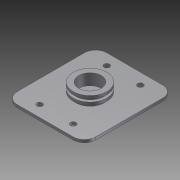
# Autodesk Inventor part: Rotation Base
Saved by Autodesk Inventor 2012 (Build 160160000, 160)
## iProperties
Created: 2011-10-21
Part Number: Rotation Base
Material: Aluminum-6061
Document SubType Name: Modeling
Designer: Tushar
Density: 2.71 g/cm^3
Mass: 90.9664 g
Surface Area: 227.283 cm^2
Volume: 33.5669 cm^3
Author: Tushar
Autodesk Inventor part; units mm, degrees
ref_plane "YZ Plane" through (0, 0, 0) normal (1, 0, 0) x (0, 1, 0)
ref_plane "XZ Plane" through (0, 0, 0) normal (0, 1, 0) x (-1, 0, 0)
ref_plane "XY Plane" through (0, 0, 0) normal (0, 0, 1) x (1, 0, 0)
sketch "Sketch2" plane through (0, 0, 0) normal (0, 1, 0) x (-1, 0, 0)
  line L0 (-44.45, 50.8) -> (44.45, 50.8)
  line L1 (44.45, 50.8) -> (44.45, -50.8)
  line L2 (44.45, -50.8) -> (-44.45, -50.8)
  line L3 (-44.45, -50.8) -> (-44.45, 50.8)
  point P0 (0, 0)
  dimension "d0" = 44.45
  dimension "d1" = 44.45
  dimension "d2" = 50.8
  dimension "d3" = 50.8
  constraints: 8 end point, 2 parallel, 1 horizontal, 1 perpendicular
  measures "d0" distance from line of L1 point (0, 0)
  measures "d1" distance from line of L3 point (0, 0)
  measures "d2" distance from line of L2 point (0, 0)
  measures "d3" distance from line of L0 point (0, 0)
extrude "Extrusion1" add sketch "Sketch2" along normal blind 3.175
fillet "Fillet1" radius 12.7 4 edges at (44.45, 1.5875, 50.8) (44.45, 1.5875, -50.8) (-44.45, 1.5875, 50.8) (-44.45, 1.5875, -50.8)
sketch "Sketch3" plane through (0, 3.175, 0) normal (0, 1, 0) x (1, 0, 0)
  line L0 (-44.45, -38.1) -> (-44.45, 38.1) projected
  line L1 (31.75, -50.8) -> (-31.75, -50.8) projected
  line L2 (44.45, 38.1) -> (44.45, -38.1) projected
  line L3 (-31.75, 50.8) -> (31.75, 50.8) projected
  point P0 (0, 0)
  point P1 (0, 0)
  point P2 (-19.05, 38.1)
  point P3 (19.05, 38.1)
  point P4 (19.05, -38.1)
  point P5 (-19.05, -38.1)
  dimension "d7" = 12.7
  dimension "d8" = 25.4
  dimension "d9" = 12.7
  dimension "d10" = 25.4
  constraints: 2 horizontal alignment, 2 vertical alignment, 1 coincident
  measures "d7" distance from line of L3 point (-19.05, 38.1)
  measures "d8" distance from line of L0 point (-19.05, 38.1)
  measures "d9" distance from line of L1 point (-19.05, -38.1)
  measures "d10" distance from line of L2 point (19.05, 38.1)
hole "Hole1" at (0, 3.175, 0) at (-19.05, 3.175, -38.1) at (19.05, 3.175, -38.1) at (19.05, 3.175, 38.1) at (-19.05, 3.175, 38.1) direction (0, -1, 0) diameter 6.35 end through all
sketch "Sketch4" plane through (0, 0, 0) normal (0, 0, 1) x (1, 0, 0)
  line L0 (12.7, 3.175) -> (12.7, 15.875)
  line L1 (12.7, 15.875) -> (19.05, 15.875)
  line L2 (19.05, 15.875) -> (19.05, 12.7)
  line L3 (19.05, 12.7) -> (15.875, 12.7)
  line L4 (15.875, 3.175) -> (12.7, 3.175)
  line L5 (15.875, 3.175) -> (12.7, 3.175)
  line L6 (15.875, 12.7) -> (15.875, 9.525)
  line L7 (15.875, 9.525) -> (19.05, 9.525)
  line L8 (19.05, 9.525) -> (19.05, 6.35)
  line L9 (19.05, 6.35) -> (15.875, 6.35)
  line L10 (15.875, 6.35) -> (15.875, 3.175)
  line L11 (15.875, 3.175) -> (12.7, 3.175)
  line L12 (0, -3.175) -> (0, 19.05) projected
  point P0 (0, 0)
  dimension "d18" = 12.7
  dimension "d19" = 6.35
  dimension "d20" = 3.175
  dimension "d21" = 3.175
  dimension "d22" = 9.525
  dimension "d23" = 12.7
  dimension "d24" = 3.175
  dimension "d25" = 3.175
  dimension "d26" = 3.175
  dimension "d27" = 3.175
  dimension "d28" = 3.175
  constraints: 24 end point, 4 parallel, 3 perpendicular, 2 collinear, 1 vertical
  measures "d18" distance of L0.start L0.end
  measures "d19" distance of L0.end L1.end
  measures "d20" distance of L1.end L2.end
  measures "d21" distance of L2.end L3.end
  measures "d22" distance of L3.end L4.start
  measures "d23" horizontal distance of L0.start point (0, 0)
  measures "d24" vertical distance of L0.start point (0, 0)
  measures "d25" distance of L3.end L6.end
  measures "d26" distance of L6.end L7.end
  measures "d27" distance of L7.end L8.end
  measures "d28" distance of L8.end L9.end
revolve "Revolution1" add sketch "Sketch4" angle 360 about axis through (0, -10, 0) along (0, 1, 0)
equation "\"d1\" = d0"
equation "\"d3\" = d2"
equation "\"d4\" = metalThickness"
equation "\"metalThickness\" = 3.175"
body "Solid1"
